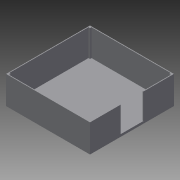
# Autodesk Inventor part: dol_obodowy_110x110
Saved by Autodesk Inventor 2015 SP1 (Build 190203100, 203)
## iProperties
Created: 2015-05-10
Part Number: dol_obodowy_110x110
Material: Ogólny
Document SubType Name: Modeling
Designer: Kuba
Density: 1 g/cm^3
Appearance: Domyślna
Author: Kuba
Autodesk Inventor part; units mm, degrees
ref_plane "YZ Plane" through (0, 0, 0) normal (1, 0, 0) x (0, 1, 0)
ref_plane "XZ Plane" through (0, 0, 0) normal (0, 1, 0) x (-1, 0, 0)
ref_plane "XY Plane" through (0, 0, 0) normal (0, 0, 1) x (1, 0, 0)
sketch "Szkic1" plane through (0, 0, 0) normal (0, 0, 1) x (1, 0, 0)
  line L0 (0, 0) -> (110, 0)
  line L1 (110, 0) -> (110, 110)
  line L2 (110, 110) -> (0, 110)
  line L3 (0, 110) -> (0, 0)
  line L4 (0, 0) -> (1, 0) construction
  line L5 (1, 0) -> (1, 1) construction
  line L6 (1, 1) -> (109, 1)
  line L7 (109, 1) -> (109, 109)
  line L8 (109, 109) -> (1, 109)
  line L9 (1, 109) -> (1, 1)
  line L10 (0, 110) -> (110, 0) construction
  line L11 (0, 0) -> (109, 109) construction
  point P0 (54.5, 54.5)
  dimension "d0" = 110
  dimension "d1" = 110
  dimension "d2" = 1
  dimension "d3" = 1
  dimension "d4" = 108
  dimension "d5" = 108
  constraints: 24 end point, 4 parallel, 3 perpendicular, 2 horizontal, 1 midpoint, 1 point on line
  measures "d0" distance of L2.end L1.end
  measures "d1" distance of L1.end L0.end
  measures "d2" distance of L0.start L4.end
  measures "d3" distance of L4.end L5.end
  measures "d4" distance of L8.end L7.end
  measures "d5" distance of L7.end L6.end
extrude "Wyciągnięcie proste1" add sketch "Szkic1" along normal blind 1.5 contours L3 L2 L1 L0 | L9 L8 L7 L6
sketch "Szkic2" plane through (0, 0, 1.5) normal (0, 0, 1) x (1, 0, 0)
  line L0 (3, 3) -> (110, 110)
  line L1 (3, 1) -> (107, 1)
  line L2 (109, 3) -> (109, 107)
  line L3 (107, 109) -> (3, 109)
  line L4 (1, 107) -> (1, 3)
  line L5 (3, 3) -> (109, 109) construction
  line L6 (109, 1) -> (1, 109) construction
  line L7 (0, 0) -> (110, 0)
  line L8 (110, 0) -> (110, 110)
  line L9 (110, 110) -> (0, 110)
  line L10 (0, 110) -> (0, 0)
  line L11 (0, 0) -> (107, 107) construction
  line L12 (107, 3) -> (0, 110) construction
  line L13 (3, 110) -> (3, 107)
  line L14 (3, 107) -> (0, 107)
  line L15 (-3, 113) -> (0, 110) construction
  line L16 (3, 113) -> (-3, 107) construction
  line L17 (1, 113) -> (3, 113)
  line L18 (0, 3) -> (3, 3)
  line L19 (3, 3) -> (3, 0)
  line L20 (107, 0) -> (107, 3)
  line L21 (107, 3) -> (110, 3)
  line L22 (110, 107) -> (107, 107)
  line L23 (107, 107) -> (107, 110)
  line L24 (3, 107) -> (107, 3)
  line L25 (109, 1) -> (110, 0)
  point P0 (0, 0)
  point P1 (0, 110)
  point P2 (55, 55)
  point P3 (55, 55)
  point P4 (55, 55)
  dimension "d8" = 108
  dimension "d9" = 108
  dimension "d10" = 110
  dimension "d11" = 110
  dimension "d14" = 6
  dimension "d17" = 360
  constraints: 53 end point, 15 point on line, 5 parallel, 4 midpoint, 3 horizontal, 3 perpendicular, 1 coincident, 29 other
  measures "d8" distance of L6.end L5.end
  measures "d9" distance of L5.end L6.start
  measures "d10" distance of L9.end L0.end
  measures "d11" distance of L0.end L7.end
  measures "d14" distance of L13.end L16.start
extrude "Wyciągnięcie proste3" add sketch "Szkic2" along normal blind 35 contours L23 L9 L0 | L0 L8 L22 | L22 L8 L21 L2 | L3 L13 L9 L23 | L19 L7 L10 L18 | L14 L10 L9 L13 | L21 L8 L7 L20 | L18 L10 L14 L4 | L1 L20 L7 L19
sketch "Szkic3" plane through (110, 0, 0) normal (1, 0, 0) x (0, 0, -1)
  line L0 (0, 0) -> (0, 40)
  line L1 (0, 0) -> (0, 110) projected
  line L2 (0, 110) -> (0, 70)
  line L3 (0, 40) -> (-36.5, 40)
  line L4 (-36.5, 40) -> (-36.5, 70)
  line L5 (-36.5, 70) -> (0, 70)
  line L6 (0, 70) -> (0, 40)
  line L7 (0, 70) -> (-3, 70)
  line L8 (-3, 70) -> (-3, 40)
  point P0 (-36.5, 109)
  dimension "d21" = 40
  dimension "d22" = 40
  dimension "d23" = 3
  constraints: 16 end point, 4 point on line, 2 parallel, 2 perpendicular, 1 horizontal
  measures "d21" distance of L0.start L0.end
  measures "d22" distance of L1.end L2.end
  measures "d23" distance of L5.end L7.end
extrude "Wyciągnięcie proste4" cut sketch "Szkic3" against normal blind 35 contours L3 L4 L5 L8
